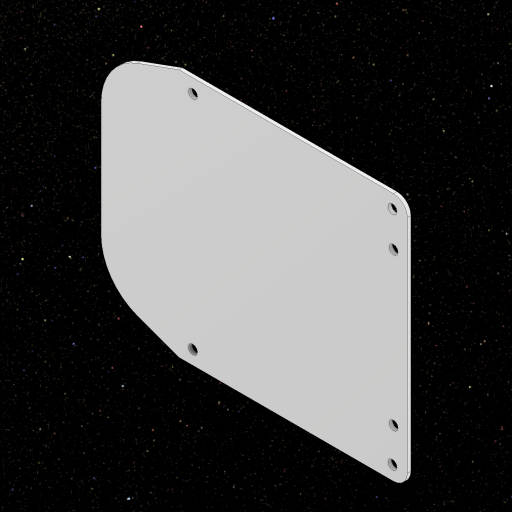
# Autodesk Inventor part: ramp
Saved by Autodesk Inventor 2024 (Build 280153000, 153)
## iProperties
Created: 2024-02-16
Part Number: ramp
Material: Acetal Resin, White
Document SubType Name: Modeling
Designer: Averey Ku
Density: 1.425 g/cm^3
Appearance: Smooth - White
Author: Averey Ku
Autodesk Inventor part; units mm, degrees
ref_plane "YZ Plane" through (0, 0, 0) normal (1, 0, 0) x (0, 1, 0)
ref_plane "XZ Plane" through (0, 0, 0) normal (0, 1, 0) x (-1, 0, 0)
ref_plane "XY Plane" through (0, 0, 0) normal (0, 0, 1) x (1, 0, 0)
sketch "Sketch1" plane through (0, 0, 0) normal (0, 0, 1) x (1, 0, 0)
  circle A0 centre (0, 0) radius 2.0955
  circle A1 centre (91.581, 0) radius 2.0955
  circle A2 centre (0, 101.6) radius 2.0955
  circle A3 centre (91.581, 101.6) radius 2.0955
  line L0 (-6.35, -6.35) -> (92.075, -6.35)
  line L1 (98.425, 0) -> (98.425, 101.6)
  line L2 (92.075, 107.95) -> (-6.35, 107.95)
  line L3 (-6.35, 107.95) -> (-25.4396, 101.002)
  line L4 (-6.35, -6.35) -> (-25.4396, 0.598)
  line L5 (-6.35, -6.35) -> (13.9647, -6.35) construction
  line L6 (-42.1523, 24.4662) -> (-42.1523, 77.1338)
  arc A4 (-25.4396, 101.002) -> (-42.1523, 77.1338) centre (-16.7523, 77.1338) ccw
  arc A5 (-42.1523, 24.4662) -> (-25.4396, 0.598) centre (-16.7523, 24.4662) ccw
  arc A6 (98.425, 101.6) -> (92.075, 107.95) centre (92.075, 101.6) ccw
  arc A7 (92.075, -6.35) -> (98.425, 0) centre (92.075, 0) ccw
  circle A8 centre (92.075, 85.725) radius 2.0955
  circle A9 centre (92.075, 15.875) radius 2.0955
  point P0 (98.425, -6.35)
  point P1 (98.425, 107.95)
  point P2 (-42.1523, 94.919)
  point P3 (-42.1523, 6.681)
  dimension "d0" = 4.191
  dimension "d1" = 4.191
  dimension "d2" = 4.191
  dimension "d3" = 4.191
  dimension "d4" = 104.775
  dimension "d5" = 114.3
  dimension "d6" = 38.1
  dimension "d7" = 160
  dimension "d8" = 38.1
  dimension "d9" = 160
  dimension "d10" = 25.4
  dimension "d11" = 6.35
  dimension "d12" = 4.191
  dimension "d13" = 4.191
  constraints: 14 end point, 10 centre point, 8 point on circle, 8 point on line, 8 tangent, 2 equal radius, 2 horizontal, 2 perpendicular, 1 coincident, 1 equal length, 1 vertical
  measures "d0" diameter of A0
  measures "d1" diameter of A1
  measures "d2" diameter of A2
  measures "d3" diameter of A3
  measures "d4" distance of L0.start point (98.425, -6.35)
  measures "d5" distance of point (98.425, -6.35) point (98.425, 107.95)
  measures "d6" distance of L2.end point (-42.152, 94.919)
  measures "d7" angle of L3 L2
  measures "d8" distance of L0.start point (-42.152, 6.681)
  measures "d9" angle of L5 L4
  measures "d10" radius of A4
  measures "d11" radius of A6
  measures "d12" diameter of A8
  measures "d13" diameter of A9
extrude "Extrusion1" add sketch "Sketch1" along normal blind 1.5875
body "Solid1"
